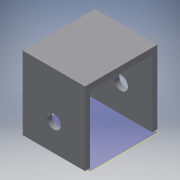
# Autodesk Inventor part: Part132
Saved by Autodesk Inventor 2016 (Build 200138000, 138)
## iProperties
Created: 2015-11-14
Part Number: Part132
Material: Generic
Document SubType Name: Modeling
Designer: jesse
Density: 1 g/cm^3
Appearance: Default
Author: jesse
Autodesk Inventor part; units mm, degrees
ref_plane "YZ Plane" through (0, 0, 0) normal (1, 0, 0) x (0, 1, 0)
ref_plane "XZ Plane" through (0, 0, 0) normal (0, 1, 0) x (-1, 0, 0)
ref_plane "XY Plane" through (0, 0, 0) normal (0, 0, 1) x (1, 0, 0)
ref_plane "Work Plane1" through (13.7597, -5.7182, -8.0415) normal (0, -1, 0) x (1, 0, 0)
sketch "Sketch1" plane through (13.7597, -5.7182, -8.0415) normal (0, -1, 0) x (1, 0, 0)
  line L0 (8.0899, -8.0899) -> (8.0899, 8.0899) construction
  line L1 (8.0899, 8.0899) -> (-8.0899, 8.0899) construction
  line L2 (-8.0899, 8.0899) -> (-8.0899, -8.0899) construction
  line L3 (-8.0899, -8.0899) -> (8.0899, -8.0899) construction
  line L4 (8.0899, 8.0899) -> (-8.0899, 8.0899)
  line L5 (-8.0899, 8.0899) -> (-8.0899, 9.3894)
  line L6 (-8.0899, 9.3894) -> (8.0899, 9.3894)
  line L7 (8.0899, 9.3894) -> (8.0899, 8.0899)
  line L8 (8.0899, -8.0899) -> (-8.0899, -8.0899)
  line L9 (-8.0899, -8.0899) -> (-8.0899, -9.3894)
  line L10 (-8.0899, -9.3894) -> (8.0899, -9.3894)
  line L11 (8.0899, -9.3894) -> (8.0899, -8.0899)
  point P0 (-13.7597, 8.0415)
  constraints: 16 end point, 4 parallel, 2 horizontal, 2 perpendicular, 1 collinear, 1 point on line
extrude "Extrusion1" add sketch "Sketch1" against normal blind 17.4625
sketch "Sketch2" plane through (21.8496, -5.7182, -17.4309) normal (0, 0, -1) x (-1, 0, 0)
  circle A0 centre (8.0899, 7.0866) radius 1.7859 projected
  point P0 (21.8496, 5.7182)
extrude "Extrusion2" cut sketch "Sketch2" against normal through all
sketch "Sketch3" plane through (13.7597, 11.7443, -8.0415) normal (0, 1, 0) x (1, 0, 0)
  line L0 (-8.0899, -9.3894) -> (8.0899, -9.3894) construction
  line L1 (-8.0899, -8.0899) -> (-8.0899, -9.3894) construction
  line L2 (8.0899, 9.3894) -> (-8.0899, 9.3894) construction
  line L3 (8.0899, 8.0899) -> (8.0899, 9.3894) construction
  line L4 (-8.0899, -9.3894) -> (8.0899, -9.3894)
  line L5 (8.0899, -9.3894) -> (8.0899, 9.3894)
  line L6 (8.0899, 9.3894) -> (-8.0899, 9.3894)
  line L7 (-8.0899, 9.3894) -> (-8.0899, -9.3894)
  point P0 (-13.7597, -8.0415)
  constraints: 8 end point, 2 parallel, 1 horizontal, 1 perpendicular
extrude "Extrusion3" add sketch "Sketch3" along normal blind 1.5875
body "Solid1"
